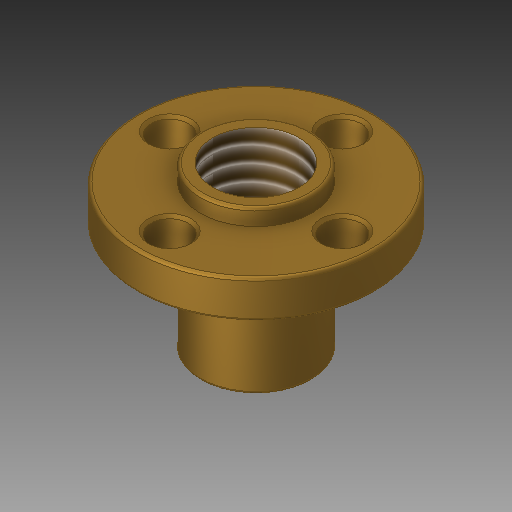
# Autodesk Inventor part: TR8 Leadscrew Nut
Saved by Autodesk Inventor 2019 (Build 230136000, 136)
## iProperties
Created: 2018-10-13
Part Number: TR8 Leadscrew Nut
Material: Brass, Soft Yellow
Document SubType Name: Modeling
Designer: Ax
Density: 8.47 g/cm^3
Appearance: Brass - Satin
Mass: 11.8229 g
Surface Area: 16.9972 cm^2
Volume: 1.39586 cm^3
Author: Ax
Autodesk Inventor part; units mm, degrees
ref_plane "YZ Plane" through (0, 0, 0) normal (1, 0, 0) x (0, 1, 0)
ref_plane "XZ Plane" through (0, 0, 0) normal (0, 1, 0) x (-1, 0, 0)
ref_plane "XY Plane" through (0, 0, 0) normal (0, 0, 1) x (1, 0, 0)
sketch "Sketch1" plane through (0, 0, 0) normal (0, 0, 1) x (1, 0, 0)
  line L0 (4, 7.5) -> (4, -7.5)
  line L1 (4, -7.5) -> (5.15, -7.5)
  line L2 (5.15, -7.5) -> (5.15, 2.5)
  line L3 (5.15, 2.5) -> (11, 2.5)
  line L4 (11, 2.5) -> (11, 6)
  line L5 (11, 6) -> (5.15, 6)
  line L6 (5.15, 6) -> (5.15, 7.5)
  line L7 (5.15, 7.5) -> (4, 7.5)
  line L8 (0, 0) -> (22.0974, 0) construction
  line L9 (0, -10.5) -> (0, 10.5) projected
  dimension "d1" = 3.5
  dimension "d2" = 1.5
  dimension "d3" = 15
  dimension "d4" = 11
  dimension "d5" = 4
  dimension "d6" = 5.15
  constraints: 18 end point, 5 perpendicular, 1 coincident, 1 collinear, 1 horizontal, 1 symmetric about line, 1 vertical
  measures "d1" distance of L3.end L4.end
  measures "d2" distance of L5.end L6.end
  measures "d3" distance between parallel lines of L1 L7
  measures "d4" horizontal distance of point (0, 0) L3.end
  measures "d5" distance from line of point (0, 0) L0
  measures "d6" horizontal distance of point (0, 0) L1.end
revolve "Revolution1" add sketch "Sketch1" angle 360 about axis through (0, -10, 0) along (0, 1, 0)
sketch "Sketch2" plane through (0, 6, 0) normal (0, 1, 0) x (1, 0, 0)
  circle A0 centre (0, 0) radius 8 construction
  line L0 (8, 0) -> (-8, 0) construction
  line L1 (0, -8) -> (0, 8) construction
  circle A1 centre (-8, 0) radius 1.75
  circle A2 centre (0, 8) radius 1.75
  circle A3 centre (8, 0) radius 1.75
  circle A4 centre (0, -8) radius 1.75
  dimension "d8" = 16
  dimension "d9" = 3.5
  constraints: 5 centre point, 5 coincident, 4 end point, 4 point on circle, 3 equal radius, 3 midpoint, 1 horizontal, 1 vertical
  measures "d8" diameter of A0
  measures "d9" diameter of A1
extrude "Extrusion1" cut sketch "Sketch2" against normal through all
chamfer "Chamfer1" distance 0.25 angle 45 4 edges at (-1.75, 6, 8) (6.25, 6, 0) (-1.75, 6, -8) (-9.75, 6, 0)
fillet "Fillet1" radius 0.25 4 edges at (-11, 6, 0) (-11, 2.5, 0) (-5.15, 7.5, 0) (-5.15, -7.5, 0)
thread "Thread1" size "TR8x1.5" class "7H" standard "ISO Metric Trapezoidal Threads" full length
body "Solid1"
